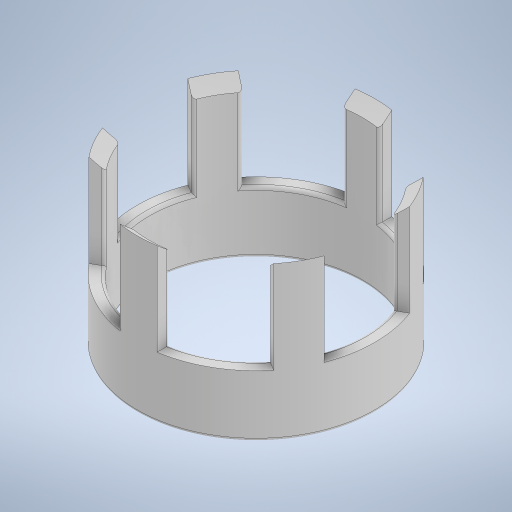
# Autodesk Inventor part: 다단로켓벨브2
Saved by Autodesk Inventor 2023 (Build 270158000, 158)
## iProperties
Created: 2023-08-25
Part Number: 다단로켓벨브2
Material: 일반
Document SubType Name: Modeling
Designer: rlatk
Density: 1 g/cm^3
Appearance: 기본값
Author: rlatk
Autodesk Inventor part; units mm, degrees
ref_plane "YZ Plane" through (0, 0, 0) normal (1, 0, 0) x (0, 1, 0)
ref_plane "XZ Plane" through (0, 0, 0) normal (0, 1, 0) x (-1, 0, 0)
ref_plane "XY Plane" through (0, 0, 0) normal (0, 0, 1) x (1, 0, 0)
sketch "스케치1" plane through (0, 0, 0) normal (0, 1, 0) x (-1, 0, 0)
  circle A0 centre (0, 0) radius 17.3
  circle A1 centre (0, 0) radius 19.3
  dimension "d0" = 34.6
  dimension "d1" = 2
  constraints: 2 centre point, 1 coincident
  measures "d0" diameter of A0
  measures "d1" radial gap between concentric circles of A0 A1
extrude "돌출1" add sketch "스케치1" along normal blind 10
sketch "스케치2" plane through (0, 10, 0) normal (0, 1, 0) x (1, 0, 0)
  line L0 (-3, -17.058641) -> (-3, -19.065414)
  line L1 (-3, 19.065414) -> (-3, 17.058641)
  circle A0 centre (0, 0) radius 19.3
  circle A1 centre (0, 0) radius 17.3
  line L2 (3, -19.065414) -> (3, -17.058641)
  line L3 (3, 17.058641) -> (3, 19.065414)
  line L4 (-3, -19.065414) -> (-3, -17.037899)
  line L5 (-3, 17.037899) -> (-3, 19.065414)
  line L6 (3, -19.065414) -> (3, -17.037899)
  line L7 (3, 17.037899) -> (3, 19.065414)
  arc A2 (-1.5, -19.241622) -> (3, -19.065414) centre (0, 0) ccw
  arc A3 (3, 19.065414) -> (-1.5, 19.241622) centre (0, 0) ccw
  arc A4 (-1.5, -17.234848) -> (3, -17.037899) centre (0, 0) ccw
  arc A5 (3, 17.037899) -> (-1.5, 17.234848) centre (0, 0) ccw
  arc A6 (-3, -19.065414) -> (3, -19.065414) centre (0, 0) ccw
  arc A7 (3, 19.065414) -> (-3, 19.065414) centre (0, 0) ccw
  arc A8 (-3, -17.037899) -> (3, -17.037899) centre (0, 0) ccw
  arc A9 (3, 17.037899) -> (-3, 17.037899) centre (0, 0) ccw
  point P0 (1.5, 17.234848)
  point P1 (1.5, -17.234848)
  constraints: 20 point on circle, 16 end point, 8 centre point, 5 vertical, 4 coincident
sketch "스케치6" plane through (0, 0, 0) normal (1, 0, 0) x (0, 1, 0)
  line L0 (0, 19.3) -> (10, 19.3)
  line L1 (25, 19.3) -> (27.217895, 19.3) construction
  line L2 (23.574365, 17.600994) -> (23.560731, 17.584746)
  line L3 (10, 17.3) -> (0, 17.3)
  arc A0 (25, 19.3) -> (23.342764, 17.3) centre (46.479094, -0.184572) ccw
  line L4 (-9.295819, 0) -> (55.774912, 0)
  line L5 (23.342764, 17.3) -> (25, 17.3)
  line L6 (25, 17.3) -> (25, 19.3)
  point P0 (0, 0)
  dimension "d13" = 58
  constraints: 8 end point, 3 point on circle, 2 horizontal, 2 point on line, 1 centre point, 1 perpendicular
  measures "d13" diameter of A0
extrude "돌출3" add sketch "스케치2" along normal blind 15 contours L4 A1 L6 L2 A0 L0 | A0 L3 L7 A1 L5 L1
revolve "회전2" cut sketch "스케치6" angle 360 about axis through (0, -10, 0) along (0, 1, 0)
pattern_circular "원형 패턴2" count 6 over 360 about axis through (0, -10, 0) along (0, 1, 0) of "돌출3", "회전2"
fillet "모깎기3" radius 0.5 21 edges at (19.3, 0, 0) (17.3, 0, 0) (17.3, 10, 0) (8.65, 10, -14.9822) (-8.65, 10, -14.9822) (-17.0368, 10, -3.0062) (-17.0368, 10, 3.0062) (-8.65, 10, 14.9822) (8.65, 10, 14.9822) (3, 16.6714, 17.0379) (-13.2553, 16.6714, 11.117) (-16.2553, 16.6714, 5.9209) (-16.2553, 16.6714, -5.9209) (-13.2553, 16.6714, -11.117) (-3, 16.6714, -17.0379) (3, 16.6714, -17.0379) (13.2553, 16.6714, -11.117) (16.2553, 16.6714, -5.9209) (16.2553, 16.6714, 5.9209) (13.2553, 16.6714, 11.117) (-3, 16.6714, 17.0379)
